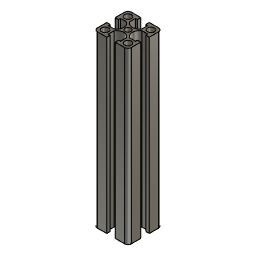
프로파일 v2 (Autodesk Fusion 360 design; units mm, degrees)
Autodesk Fusion 360 part; units mm, degrees
sketch "스케치1" plane through (0, 0, 0) normal (0, 0, 1) x (1, 0, 0)
  circle A0 centre (-13.5, 13.5) radius 4
  circle A1 centre (13.5, 13.5) radius 4
  circle A2 centre (-13.5, -13.5) radius 4
  circle A3 centre (13.5, -13.5) radius 4
  line L0 (17.5, -13.5) -> (20, -13.5)
  circle A4 centre (0, 0) radius 3.4
  line L1 (20, 16) -> (20, 5)
  line L2 (20, -5) -> (20, -16)
  arc A5 (-9.0629, -7.25) -> (-9.0629, 7.25) centre (-13.5, 0) ccw
  line L3 (-20, -16) -> (-20, -5)
  line L4 (-20, 5) -> (-20, 16)
  line L5 (-16, 20) -> (-5, 20)
  line L6 (5, 20) -> (16, 20)
  line L7 (16, -20) -> (5, -20)
  line L8 (-5, -20) -> (-16, -20)
  line L9 (-5, -16) -> (-5, -20)
  line L10 (5, -16) -> (5, -20)
  line L11 (5, -16) -> (7.25, -16)
  line L12 (-7.25, -16) -> (-5, -16)
  arc A6 (7.25, -9.0629) -> (-7.25, -9.0629) centre (0, -13.5) ccw
  line L13 (-7.25, -9.0629) -> (-7.25, -16)
  line L14 (-20, 5) -> (-16, 5)
  line L15 (-20, -5) -> (-16, -5)
  line L16 (-16, -5) -> (-16, -7.25)
  line L17 (-16, 7.25) -> (-16, 5)
  line L18 (-16, -7.25) -> (-9.0629, -7.25)
  line L19 (7.25, -9.0629) -> (7.25, -16)
  arc A7 (-7.25, 9.0629) -> (7.25, 9.0629) centre (0, 13.5) ccw
  line L20 (5, 16) -> (5, 20)
  line L21 (16, 20) -> (5, 20)
  line L22 (20, 5) -> (20, 16)
  line L23 (-7.25, 9.0629) -> (-7.25, 16)
  line L24 (5, 16) -> (7.25, 16)
  circle A8 centre (13.5, 13.5) radius 4
  line L25 (-5, 16) -> (-5, 20)
  line L26 (-20, 16) -> (-20, 5)
  line L27 (-16, 7.25) -> (-9.0629, 7.25)
  line L28 (-7.25, 16) -> (-5, 16)
  line L29 (-16, 5) -> (-16, 7.25)
  line L30 (7.25, 9.0629) -> (7.25, 16)
  line L31 (-5, 20) -> (-16, 20)
  line L32 (-20, 5) -> (-16, 5)
  circle A9 centre (-13.5, 13.5) radius 4
  line L33 (5, 20) -> (5, 16)
  line L34 (-5, 20) -> (-5, 16)
  line L35 (-16, 7.25) -> (-9.0629, 7.25)
  arc A10 (-7.25, 9.0629) -> (7.25, 9.0629) centre (0, 13.5) ccw
  line L36 (7.25, 13.5) -> (7.25, 9.0629)
  line L37 (5, 20) -> (16, 20)
  line L38 (20, -16) -> (20, -5)
  line L39 (7.25, -9.0629) -> (7.25, -16)
  line L40 (16, 5) -> (16, 7.25)
  line L41 (16, 20) -> (5, 20)
  arc A11 (9.0629, 7.25) -> (9.0629, -7.25) centre (13.5, 0) ccw
  line L42 (7.25, -16) -> (5, -16)
  line L43 (16, -5) -> (16, -7.25)
  line L44 (16, 7.25) -> (16, 5)
  line L45 (7.25, 16) -> (5, 16)
  line L46 (5, -16) -> (5, -20)
  line L47 (20, 5) -> (16, 5)
  line L48 (7.25, 9.0629) -> (7.25, 16)
  line L49 (16, -7.25) -> (9.0629, -7.25)
  line L50 (20, -5) -> (16, -5)
  circle A12 centre (13.5, 13.5) radius 4
  circle A13 centre (13.5, -13.5) radius 4
  line L51 (5, -20) -> (16, -20)
  line L52 (5, 20) -> (5, 16)
  line L53 (5, 16) -> (5, 20)
  line L54 (20, 16) -> (20, 5)
  line L55 (20, 5) -> (20, 16)
  line L56 (20, 5) -> (16, 5)
  circle A14 centre (13.5, 13.5) radius 4
  line L57 (7.25, 5.7609) -> (7.25, 5)
  line L58 (7.25, -5) -> (7.25, -5.7609)
  line L59 (6.6261, -5) -> (7.25, -5)
  line L60 (16, -5) -> (20, -5)
  line L61 (6.6261, 5) -> (7.25, 5)
  line L62 (16, 5) -> (20, 5)
  line L63 (6.6261, 5) -> (7.25, 5)
  line L64 (16, 5) -> (20, 5)
  line L65 (9.0629, 7.25) -> (16, 7.25)
  line L66 (9.0629, -7.25) -> (16, -7.25)
  arc A15 (9.0629, 7.25) -> (9.0629, -7.25) centre (13.5, 0) ccw
  arc A16 (-20, -16) -> (-16, -20) centre (-16, -16) ccw
  arc A17 (-16, 20) -> (-20, 16) centre (-16, 16) ccw
  arc A18 (20, 16) -> (16, 20) centre (16, 16) ccw
  arc A19 (16, -20) -> (20, -16) centre (16, -16) ccw
  dimension "d10" = 8
  dimension "d11" = 8
  dimension "d12" = 8
  dimension "d13" = 8
  dimension "d14" = 6.8
  dimension "d15" = 27
  dimension "d18" = 4
  dimension "d19" = 4
  dimension "d21" = 14.5
  dimension "d22" = 4
  dimension "d23" = 4
  dimension "d26" = 40
  constraint horizontal L5
  constraint vertical L1
  constraint horizontal L7
  constraint vertical L3
  constraint coincident L0.end L1
  constraint coincident A3 L0.start
  constraint coincident A4.centre origin
  constraint perpendicular L7 L34
  constraint coincident L4.start L3
  constraint tangent A5 L34
  constraint coincident L1.end L14
  constraint coincident L2.start L15
  constraint collinear L1 L2
  constraint collinear L3 L4
  constraint collinear L5 L6
  constraint coincident L7.end L33
  constraint coincident L8.start L34
  constraint collinear L7 L8
  constraint perpendicular L7 L36
  constraint collinear L9 L34
  constraint collinear L10 L33
  constraint coincident A6.start L36
  constraint perpendicular L1 L35
  constraint perpendicular L2 L18
  constraint collinear L14 L63
  constraint collinear L15 L59
  constraint collinear L19 L36
  constraint collinear L36 L57
  constraint collinear L57 L58
  constraint collinear L59 L60
  constraint collinear L61 L62
  constraint collinear L63 L64
  constraint tangent L3 A16
  constraint tangent L8 A16
  constraint tangent L26 A17
  constraint tangent L31 A17
  constraint tangent L37 A18
  constraint tangent L22 A18
  constraint equal A17 A18
  constraint tangent L2 A19
  constraint tangent L51 A19
  constraint equal A17 A19
  measures "d10" diameter of A0
  measures "d11" diameter of A1
  measures "d12" diameter of A2
  measures "d13" diameter of A3
  measures "d14" diameter of A4
  measures "d15" distance of A1.centre A3.centre
  measures "d18" distance of L7 L11
  measures "d19" distance of L8 L12
  measures "d21" distance of L13 L36
  measures "d22" radius of A16
  measures "d23" radius of A17
  measures "d26" distance of L3.start L2.end
extrude "돌출1" add sketch "스케치1" along normal blind 200 contours L1 L2 A5 L3 L4 L5 L6 L7 L8 L9 L10 L11 L12 A6 L13 L14 L15 L16 L17 L18 L19 A7 L20 L21 L22 L23 L24 L25 L26 L27 L28 L29 L30 L31 L32 L33 L34 L35 A10 L36 L37 L38 L39 L40 L41 A11 L42 L43 L44 L45 L46 L47 L48 L49 L50 L51 L52 L53 L54 L55 L56 L60 L62 L64 L65 L66 A15 A16 A17 A18 A19
